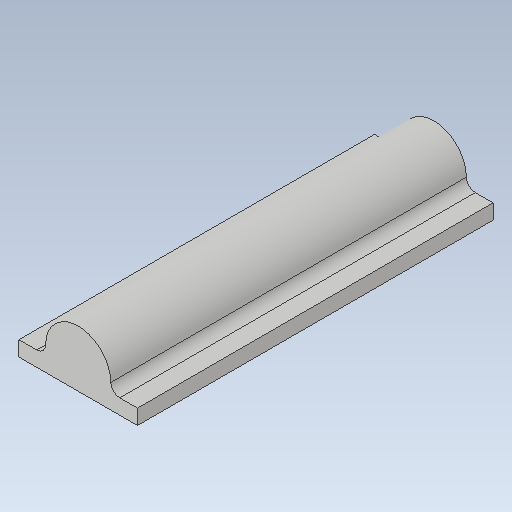
# Autodesk Inventor part: zab
Saved by Autodesk Inventor 2020 (Build 240168000, 168)
## iProperties
Created: 2020-05-17
Part Number: zab
Material: Generic
Document SubType Name: Modeling
Designer: estee
Density: 1 g/cm^3
Appearance: Default
Author: estee
Autodesk Inventor part; units mm, degrees
ref_plane "YZ Plane" through (0, 0, 0) normal (1, 0, 0) x (0, 1, 0)
ref_plane "XZ Plane" through (0, 0, 0) normal (0, 1, 0) x (-1, 0, 0)
sketch "Sketch1" plane through (0, 0, 0) normal (0, 0, 1) x (1, 0, 0)
  arc A0 (0.55, 0) -> (-0.55, 0) centre (0, 0) ccw
  arc A1 (0.55, 0) -> (0.7, -0.15) centre (0.7, 0) ccw
  arc A2 (-0.7, -0.15) -> (-0.55, 0) centre (-0.7, 0) ccw
  line L0 (0.7, -0.15) -> (1, -0.15)
  line L1 (-0.7, -0.15) -> (-1, -0.15)
  line L2 (-1, -0.15) -> (-1, -0.404)
  line L3 (-1, -0.404) -> (1, -0.404)
  line L4 (1, -0.404) -> (1, -0.15)
  dimension "d4" = 0.3
  dimension "d5" = 0.3
  dimension "d6" = 0
  dimension "d7" = 0
  dimension "d8" = 0.3
  dimension "d9" = 0.3
  dimension "d10" = 0.254
  constraints: 10 end point, 6 point on circle, 3 centre point, 2 horizontal, 2 perpendicular, 1 tangent, 1 vertical
  measures "d4" diameter of A1
  measures "d5" diameter of A2
  measures "d6" vertical distance between centres of A0 A1
  measures "d7" vertical distance between centres of A0 A2
  measures "d8" distance of L0.start L0.end
  measures "d9" distance of L1.start L1.end
  measures "d10" distance of L1.end L2.end
extrude "Extrusion1" add sketch "Sketch1" along normal blind 6
ref_plane "Work Plane1" through (-1, -0.404, 0) normal (0, -1, 0) x (1, 0, 0)
sketch "Sketch2" plane through (-1, -0.404, 0) normal (0, -1, 0) x (1, 0, 0)
  line L0 (2, 0) -> (0, 0) projected
  line L1 (0, 0) -> (0, 6) projected
  point P0 (1, 0)
  point P1 (1, 3)
  dimension "d14" = 3
  dimension "d15" = 1
  measures "d14" distance from line of L0 point (1, 3)
  measures "d15" distance from line of L1 point (1, 3)
body "Solid1"
